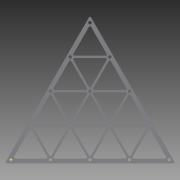
# Autodesk Inventor part: grid16-top
Saved by Autodesk Inventor 2013 (Build 170138000, 138)
## iProperties
Created: 2013-03-05
Part Number: grid16-top
Material: Generic
Document SubType Name: Modeling
Designer: Beth Scott
Density: 1 g/cm^3
Author: Beth Scott
Autodesk Inventor part; units mm, degrees
ref_plane "YZ Plane" through (0, 0, 0) normal (1, 0, 0) x (0, 1, 0)
ref_plane "XZ Plane" through (0, 0, 0) normal (0, 1, 0) x (-1, 0, 0)
ref_plane "XY Plane" through (0, 0, 0) normal (0, 0, 1) x (1, 0, 0)
sketch "Triangle 1mm" plane through (0, 0, 0) normal (0, 0, 1) x (1, 0, 0)
  line L0 (0, 0) -> (16.6665, 28.8672) construction
  line L1 (16.6665, 28.8672) -> (33.333, 0) construction
  line L2 (33.333, 0) -> (0, 0) construction
  line L3 (2.5981, 2.5) -> (15.8005, 25.3672)
  line L4 (17.5325, 25.3672) -> (30.7349, 2.5)
  line L5 (29.8689, 1) -> (3.4641, 1)
  arc A0 (17.5325, 25.3672) -> (15.8005, 25.3672) centre (16.6665, 24.8672) ccw
  arc A1 (29.8689, 1) -> (30.7349, 2.5) centre (29.8689, 2) ccw
  arc A2 (2.5981, 2.5) -> (3.4641, 1) centre (3.4641, 2) ccw
  line L6 (33.333, 0) -> (8.3332, 14.4336) construction
  line L7 (0, 0) -> (24.9997, 14.4336) construction
  line L8 (16.6665, 28.8672) -> (16.6665, 0) construction
  point P0 (16.9666, 9.7956)
  dimension "d14" = 33.333
  dimension "d17" = 1
  dimension "d18" = 1
  measures "d14" distance of L1.end L0.start
  measures "d17" radius of A2
  measures "d18" distance from line of L4 L7.end
sketch "Tri16 1mm" plane through (0, 0, 0) normal (0, 0, 1) x (1, 0, 0)
  line L0 (0, 0) -> (16.6665, 28.8672) construction
  line L1 (16.6665, 28.8672) -> (33.333, 0) construction
  line L2 (33.333, 0) -> (0, 0) construction
  line L3 (2.5981, 2.5) -> (15.8005, 25.3672)
  line L4 (17.5325, 25.3672) -> (30.7349, 2.5)
  line L5 (29.8689, 1) -> (3.4641, 1)
  arc A0 (17.5325, 25.3672) -> (15.8005, 25.3672) centre (16.6665, 24.8672) ccw
  arc A1 (29.8689, 1) -> (30.7349, 2.5) centre (29.8689, 2) ccw
  arc A2 (2.5981, 2.5) -> (3.4641, 1) centre (3.4641, 2) ccw
  line L6 (33.333, 0) -> (8.3333, 14.4336) construction
  line L7 (0, 0) -> (24.9998, 14.4336) construction
  line L8 (16.6665, 28.8672) -> (16.6665, 0) construction
  line L9 (33.333, 0) -> (49.9995, 28.8672) construction
  line L10 (49.9995, 28.8672) -> (66.666, 0) construction
  line L11 (66.666, 0) -> (33.333, 0) construction
  line L12 (35.9311, 2.5) -> (49.1335, 25.3672)
  line L13 (50.8655, 25.3672) -> (64.0679, 2.5)
  line L14 (63.2019, 1) -> (36.7971, 1)
  arc A3 (50.8655, 25.3672) -> (49.1335, 25.3672) centre (49.9995, 24.8672) ccw
  arc A4 (63.2019, 1) -> (64.0679, 2.5) centre (63.2019, 2) ccw
  arc A5 (35.9311, 2.5) -> (36.7971, 1) centre (36.7971, 2) ccw
  line L15 (66.666, 0) -> (41.6663, 14.4336) construction
  line L16 (33.333, 0) -> (58.3328, 14.4336) construction
  line L17 (49.9995, 28.8672) -> (49.9995, 0) construction
  line L18 (49.9995, 28.8672) -> (33.333, 0) construction
  line L19 (33.333, 0) -> (16.6665, 28.8672) construction
  line L20 (16.6665, 28.8672) -> (49.9995, 28.8672) construction
  line L21 (47.4014, 26.3672) -> (34.199, 3.5)
  line L22 (32.467, 3.5) -> (19.2646, 26.3672)
  line L23 (20.1306, 27.8672) -> (46.5354, 27.8672)
  arc A6 (32.467, 3.5) -> (34.199, 3.5) centre (33.333, 4) ccw
  arc A7 (20.1306, 27.8672) -> (19.2646, 26.3672) centre (20.1306, 26.8672) ccw
  arc A8 (47.4014, 26.3672) -> (46.5354, 27.8672) centre (46.5354, 26.8672) ccw
  line L24 (16.6665, 28.8672) -> (41.6663, 14.4336) construction
  line L25 (49.9995, 28.8672) -> (24.9998, 14.4336) construction
  line L26 (33.333, 0) -> (33.333, 28.8672) construction
  line L27 (83.3325, 28.8672) -> (66.666, 0) construction
  line L28 (66.666, 0) -> (49.9995, 28.8672) construction
  line L29 (49.9995, 28.8672) -> (83.3325, 28.8672) construction
  line L30 (80.7344, 26.3672) -> (67.532, 3.5)
  line L31 (65.8, 3.5) -> (52.5976, 26.3672)
  line L32 (53.4636, 27.8672) -> (79.8684, 27.8672)
  arc A9 (65.8, 3.5) -> (67.532, 3.5) centre (66.666, 4) ccw
  arc A10 (53.4636, 27.8672) -> (52.5976, 26.3672) centre (53.4636, 26.8672) ccw
  arc A11 (80.7344, 26.3672) -> (79.8684, 27.8672) centre (79.8684, 26.8672) ccw
  line L33 (49.9995, 28.8672) -> (74.9993, 14.4336) construction
  line L34 (83.3325, 28.8672) -> (58.3328, 14.4336) construction
  line L35 (66.666, 0) -> (66.666, 28.8672) construction
  line L36 (66.666, 0) -> (83.3325, 28.8672) construction
  line L37 (83.3325, 28.8672) -> (99.999, 0) construction
  line L38 (99.999, 0) -> (66.666, 0) construction
  line L39 (69.2641, 2.5) -> (82.4665, 25.3672)
  line L40 (84.1985, 25.3672) -> (97.4009, 2.5)
  line L41 (96.5349, 1) -> (70.1301, 1)
  arc A12 (84.1985, 25.3672) -> (82.4665, 25.3672) centre (83.3325, 24.8672) ccw
  arc A13 (96.5349, 1) -> (97.4009, 2.5) centre (96.5349, 2) ccw
  arc A14 (69.2641, 2.5) -> (70.1301, 1) centre (70.1301, 2) ccw
  line L42 (99.999, 0) -> (74.9993, 14.4336) construction
  line L43 (66.666, 0) -> (91.6658, 14.4336) construction
  line L44 (83.3325, 28.8672) -> (83.3325, 0) construction
  line L45 (99.999, 0) -> (116.6655, 28.8672) construction
  line L46 (116.6655, 28.8672) -> (133.332, 0) construction
  line L47 (133.332, 0) -> (99.999, 0) construction
  line L48 (102.5971, 2.5) -> (115.7995, 25.3672)
  line L49 (117.5315, 25.3672) -> (130.7339, 2.5)
  line L50 (129.8679, 1) -> (103.4631, 1)
  arc A15 (117.5315, 25.3672) -> (115.7995, 25.3672) centre (116.6655, 24.8672) ccw
  arc A16 (129.8679, 1) -> (130.7339, 2.5) centre (129.8679, 2) ccw
  arc A17 (102.5971, 2.5) -> (103.4631, 1) centre (103.4631, 2) ccw
  line L51 (133.332, 0) -> (108.3323, 14.4336) construction
  line L52 (99.999, 0) -> (124.9988, 14.4336) construction
  line L53 (116.6655, 28.8672) -> (116.6655, 0) construction
  line L54 (116.6655, 28.8672) -> (99.999, 0) construction
  line L55 (99.999, 0) -> (83.3325, 28.8672) construction
  line L56 (83.3325, 28.8672) -> (116.6655, 28.8672) construction
  line L57 (114.0674, 26.3672) -> (100.865, 3.5)
  line L58 (99.133, 3.5) -> (85.9306, 26.3672)
  line L59 (86.7966, 27.8672) -> (113.2014, 27.8672)
  arc A18 (99.133, 3.5) -> (100.865, 3.5) centre (99.999, 4) ccw
  arc A19 (86.7966, 27.8672) -> (85.9306, 26.3672) centre (86.7966, 26.8672) ccw
  arc A20 (114.0674, 26.3672) -> (113.2014, 27.8672) centre (113.2014, 26.8672) ccw
  line L60 (83.3325, 28.8672) -> (108.3323, 14.4336) construction
  line L61 (116.6655, 28.8672) -> (91.6658, 14.4336) construction
  line L62 (99.999, 0) -> (99.999, 28.8672) construction
  line L63 (16.6665, 28.8672) -> (33.333, 57.7344) construction
  line L64 (33.333, 57.7344) -> (49.9995, 28.8672) construction
  line L65 (49.9995, 28.8672) -> (16.6665, 28.8672) construction
  line L66 (19.2646, 31.3672) -> (32.467, 54.2344)
  line L67 (34.199, 54.2344) -> (47.4014, 31.3672)
  line L68 (46.5354, 29.8672) -> (20.1306, 29.8672)
  arc A21 (34.199, 54.2344) -> (32.467, 54.2344) centre (33.333, 53.7344) ccw
  arc A22 (46.5354, 29.8672) -> (47.4014, 31.3672) centre (46.5354, 30.8672) ccw
  arc A23 (19.2646, 31.3672) -> (20.1306, 29.8672) centre (20.1306, 30.8672) ccw
  line L69 (49.9995, 28.8672) -> (24.9998, 43.3008) construction
  line L70 (16.6665, 28.8672) -> (41.6663, 43.3008) construction
  line L71 (33.333, 57.7344) -> (33.333, 28.8672) construction
  line L72 (33.333, 57.7344) -> (49.9995, 86.6017) construction
  line L73 (49.9995, 86.6017) -> (66.666, 57.7344) construction
  line L74 (66.666, 57.7344) -> (33.333, 57.7344) construction
  line L75 (35.9311, 60.2344) -> (49.1335, 83.1017)
  line L76 (50.8655, 83.1017) -> (64.0679, 60.2344)
  line L77 (63.2019, 58.7344) -> (36.7971, 58.7344)
  arc A24 (50.8655, 83.1017) -> (49.1335, 83.1017) centre (49.9995, 82.6017) ccw
  arc A25 (63.2019, 58.7344) -> (64.0679, 60.2344) centre (63.2019, 59.7344) ccw
  arc A26 (35.9311, 60.2344) -> (36.7971, 58.7344) centre (36.7971, 59.7344) ccw
  line L78 (66.666, 57.7344) -> (41.6663, 72.1681) construction
  line L79 (33.333, 57.7344) -> (58.3328, 72.1681) construction
  line L80 (49.9995, 86.6017) -> (49.9995, 57.7344) construction
  line L81 (49.9995, 86.6017) -> (66.666, 115.4689) construction
  line L82 (66.666, 115.4689) -> (83.3325, 86.6017) construction
  line L83 (83.3325, 86.6017) -> (49.9995, 86.6017) construction
  line L84 (52.5976, 89.1017) -> (65.8, 111.9689)
  line L85 (67.532, 111.9689) -> (80.7344, 89.1017)
  line L86 (79.8684, 87.6017) -> (53.4636, 87.6017)
  arc A27 (67.532, 111.9689) -> (65.8, 111.9689) centre (66.666, 111.4689) ccw
  arc A28 (79.8684, 87.6017) -> (80.7344, 89.1017) centre (79.8684, 88.6017) ccw
  arc A29 (52.5976, 89.1017) -> (53.4636, 87.6017) centre (53.4636, 88.6017) ccw
  line L87 (83.3325, 86.6017) -> (58.3328, 101.0353) construction
  line L88 (49.9995, 86.6017) -> (74.9993, 101.0353) construction
  line L89 (66.666, 115.4689) -> (66.666, 86.6017) construction
  line L90 (66.666, 57.7344) -> (49.9995, 28.8672) construction
  line L91 (49.9995, 28.8672) -> (33.333, 57.7344) construction
  line L92 (33.333, 57.7344) -> (66.666, 57.7344) construction
  line L93 (64.0679, 55.2344) -> (50.8655, 32.3672)
  line L94 (49.1335, 32.3672) -> (35.9311, 55.2344)
  line L95 (36.7971, 56.7344) -> (63.2019, 56.7344)
  arc A30 (49.1335, 32.3672) -> (50.8655, 32.3672) centre (49.9995, 32.8672) ccw
  arc A31 (36.7971, 56.7344) -> (35.9311, 55.2344) centre (36.7971, 55.7344) ccw
  arc A32 (64.0679, 55.2344) -> (63.2019, 56.7344) centre (63.2019, 55.7344) ccw
  line L96 (33.333, 57.7344) -> (58.3328, 43.3008) construction
  line L97 (66.666, 57.7344) -> (41.6663, 43.3008) construction
  line L98 (49.9995, 28.8672) -> (49.9995, 57.7344) construction
  line L99 (83.3325, 86.6017) -> (66.666, 57.7344) construction
  line L100 (66.666, 57.7344) -> (49.9995, 86.6017) construction
  line L101 (49.9995, 86.6017) -> (83.3325, 86.6017) construction
  line L102 (80.7344, 84.1017) -> (67.532, 61.2344)
  line L103 (65.8, 61.2344) -> (52.5976, 84.1017)
  line L104 (53.4636, 85.6017) -> (79.8684, 85.6017)
  arc A33 (65.8, 61.2344) -> (67.532, 61.2344) centre (66.666, 61.7344) ccw
  arc A34 (53.4636, 85.6017) -> (52.5976, 84.1017) centre (53.4636, 84.6017) ccw
  arc A35 (80.7344, 84.1017) -> (79.8684, 85.6017) centre (79.8684, 84.6017) ccw
  line L105 (49.9995, 86.6017) -> (74.9993, 72.1681) construction
  line L106 (83.3325, 86.6017) -> (58.3328, 72.1681) construction
  line L107 (66.666, 57.7344) -> (66.666, 86.6017) construction
  line L108 (66.666, 57.7344) -> (83.3325, 86.6017) construction
  line L109 (83.3325, 86.6017) -> (99.999, 57.7344) construction
  line L110 (99.999, 57.7344) -> (66.666, 57.7344) construction
  line L111 (69.2641, 60.2344) -> (82.4665, 83.1017)
  line L112 (84.1985, 83.1017) -> (97.4009, 60.2344)
  line L113 (96.5349, 58.7344) -> (70.1301, 58.7344)
  arc A36 (84.1985, 83.1017) -> (82.4665, 83.1017) centre (83.3325, 82.6017) ccw
  arc A37 (96.5349, 58.7344) -> (97.4009, 60.2344) centre (96.5349, 59.7344) ccw
  arc A38 (69.2641, 60.2344) -> (70.1301, 58.7344) centre (70.1301, 59.7344) ccw
  line L114 (99.999, 57.7344) -> (74.9993, 72.1681) construction
  line L115 (66.666, 57.7344) -> (91.6658, 72.1681) construction
  line L116 (83.3325, 86.6017) -> (83.3325, 57.7344) construction
  line L117 (49.9995, 28.8672) -> (66.666, 57.7344) construction
  line L118 (66.666, 57.7344) -> (83.3325, 28.8672) construction
  line L119 (83.3325, 28.8672) -> (49.9995, 28.8672) construction
  line L120 (52.5976, 31.3672) -> (65.8, 54.2344)
  line L121 (67.532, 54.2344) -> (80.7344, 31.3672)
  line L122 (79.8684, 29.8672) -> (53.4636, 29.8672)
  arc A39 (67.532, 54.2344) -> (65.8, 54.2344) centre (66.666, 53.7344) ccw
  arc A40 (79.8684, 29.8672) -> (80.7344, 31.3672) centre (79.8684, 30.8672) ccw
  arc A41 (52.5976, 31.3672) -> (53.4636, 29.8672) centre (53.4636, 30.8672) ccw
  line L123 (83.3325, 28.8672) -> (58.3328, 43.3008) construction
  line L124 (49.9995, 28.8672) -> (74.9993, 43.3008) construction
  line L125 (66.666, 57.7344) -> (66.666, 28.8672) construction
  line L126 (83.3325, 28.8672) -> (99.999, 57.7344) construction
  line L127 (99.999, 57.7344) -> (116.6655, 28.8672) construction
  line L128 (116.6655, 28.8672) -> (83.3325, 28.8672) construction
  line L129 (85.9306, 31.3672) -> (99.133, 54.2344)
  line L130 (100.865, 54.2344) -> (114.0674, 31.3672)
  line L131 (113.2014, 29.8672) -> (86.7966, 29.8672)
  arc A42 (100.865, 54.2344) -> (99.133, 54.2344) centre (99.999, 53.7344) ccw
  arc A43 (113.2014, 29.8672) -> (114.0674, 31.3672) centre (113.2014, 30.8672) ccw
  arc A44 (85.9306, 31.3672) -> (86.7966, 29.8672) centre (86.7966, 30.8672) ccw
  line L132 (116.6655, 28.8672) -> (91.6658, 43.3008) construction
  line L133 (83.3325, 28.8672) -> (108.3323, 43.3008) construction
  line L134 (99.999, 57.7344) -> (99.999, 28.8672) construction
  line L135 (99.999, 57.7344) -> (83.3325, 28.8672) construction
  line L136 (83.3325, 28.8672) -> (66.666, 57.7344) construction
  line L137 (66.666, 57.7344) -> (99.999, 57.7344) construction
  line L138 (97.4009, 55.2344) -> (84.1985, 32.3672)
  line L139 (82.4665, 32.3672) -> (69.2641, 55.2344)
  line L140 (70.1301, 56.7344) -> (96.5349, 56.7344)
  arc A45 (82.4665, 32.3672) -> (84.1985, 32.3672) centre (83.3325, 32.8672) ccw
  arc A46 (70.1301, 56.7344) -> (69.2641, 55.2344) centre (70.1301, 55.7344) ccw
  arc A47 (97.4009, 55.2344) -> (96.5349, 56.7344) centre (96.5349, 55.7344) ccw
  line L141 (66.666, 57.7344) -> (91.6658, 43.3008) construction
  line L142 (99.999, 57.7344) -> (74.9993, 43.3008) construction
  line L143 (83.3325, 28.8672) -> (83.3325, 57.7344) construction
  point P0 (66.741, 38.5329)
sketch "Top Plate" plane through (0, 0, 0) normal (0, 1, 0) x (-1, 0, 0)
  line L0 (-4.3301, -1.5) -> (65.8, 119.9689)
  line L1 (67.532, 119.9689) -> (137.6621, -1.5)
  line L2 (-3.4641, -3) -> (136.7961, -3)
  circle A0 centre (33.333, 0) radius 1.5
  circle A1 centre (0, 0) radius 1.5
  circle A2 centre (16.6665, 28.8672) radius 1.5
  circle A3 centre (33.333, 57.7344) radius 1.5
  circle A4 centre (49.9995, 28.8672) radius 1.5
  circle A5 centre (66.666, 0) radius 1.5
  circle A6 centre (99.999, 0) radius 1.5
  circle A7 centre (133.332, 0) radius 1.5
  circle A8 centre (116.6655, 28.8672) radius 1.5
  circle A9 centre (99.999, 57.7344) radius 1.5
  circle A10 centre (83.3325, 28.8672) radius 1.5
  circle A11 centre (66.666, 57.7344) radius 1.5
  circle A12 centre (83.3325, 86.6017) radius 1.5
  circle A13 centre (49.9995, 86.6017) radius 1.5
  circle A14 centre (66.666, 115.4689) radius 1.5
  arc A15 (67.532, 119.9689) -> (65.8, 119.9689) centre (66.666, 119.4689) ccw
  arc A16 (136.7961, -3) -> (137.6621, -1.5) centre (136.7961, -2) ccw
  arc A17 (-4.3301, -1.5) -> (-3.4641, -3) centre (-3.4641, -2) ccw
  line L3 (0, 0) -> (-13.8976, -8.0238) construction
  line L4 (133.332, 0) -> (144.2364, -6.2956) construction
  line L5 (17.9655, 29.6172) -> (19.2646, 30.3672) construction
  line L6 (15.3675, 29.6172) -> (14.0684, 30.3672) construction
  line L7 (0, 0) -> (16.6665, 28.8672) construction
  line L8 (16.6665, 28.8672) -> (33.333, 0) construction
  line L9 (33.333, 0) -> (0, 0) construction
  line L10 (2.5981, 2.5) -> (15.8005, 25.3672)
  line L11 (17.5325, 25.3672) -> (30.7349, 2.5)
  line L12 (29.8689, 1) -> (3.4641, 1)
  arc A18 (17.5325, 25.3672) -> (15.8005, 25.3672) centre (16.6665, 24.8672) ccw
  arc A19 (29.8689, 1) -> (30.7349, 2.5) centre (29.8689, 2) ccw
  arc A20 (2.5981, 2.5) -> (3.4641, 1) centre (3.4641, 2) ccw
  line L13 (33.333, 0) -> (8.3333, 14.4336) construction
  line L14 (0, 0) -> (24.9998, 14.4336) construction
  line L15 (16.6665, 28.8672) -> (16.6665, 0) construction
  line L16 (33.333, 0) -> (49.9995, 28.8672) construction
  line L17 (49.9995, 28.8672) -> (66.666, 0) construction
  line L18 (66.666, 0) -> (33.333, 0) construction
  line L19 (35.9311, 2.5) -> (49.1335, 25.3672)
  line L20 (50.8655, 25.3672) -> (64.0679, 2.5)
  line L21 (63.2019, 1) -> (36.7971, 1)
  arc A21 (50.8655, 25.3672) -> (49.1335, 25.3672) centre (49.9995, 24.8672) ccw
  arc A22 (63.2019, 1) -> (64.0679, 2.5) centre (63.2019, 2) ccw
  arc A23 (35.9311, 2.5) -> (36.7971, 1) centre (36.7971, 2) ccw
  line L22 (66.666, 0) -> (41.6663, 14.4336) construction
  line L23 (33.333, 0) -> (58.3328, 14.4336) construction
  line L24 (49.9995, 28.8672) -> (49.9995, 0) construction
  line L25 (49.9995, 28.8672) -> (33.333, 0) construction
  line L26 (33.333, 0) -> (16.6665, 28.8672) construction
  line L27 (16.6665, 28.8672) -> (49.9995, 28.8672) construction
  line L28 (47.4014, 26.3672) -> (34.199, 3.5)
  line L29 (32.467, 3.5) -> (19.2646, 26.3672)
  line L30 (20.1306, 27.8672) -> (46.5354, 27.8672)
  arc A24 (32.467, 3.5) -> (34.199, 3.5) centre (33.333, 4) ccw
  arc A25 (20.1306, 27.8672) -> (19.2646, 26.3672) centre (20.1306, 26.8672) ccw
  arc A26 (47.4014, 26.3672) -> (46.5354, 27.8672) centre (46.5354, 26.8672) ccw
  line L31 (16.6665, 28.8672) -> (41.6663, 14.4336) construction
  line L32 (49.9995, 28.8672) -> (24.9998, 14.4336) construction
  line L33 (33.333, 0) -> (33.333, 28.8672) construction
  line L34 (83.3325, 28.8672) -> (66.666, 0) construction
  line L35 (66.666, 0) -> (49.9995, 28.8672) construction
  line L36 (49.9995, 28.8672) -> (83.3325, 28.8672) construction
  line L37 (80.7344, 26.3672) -> (67.532, 3.5)
  line L38 (65.8, 3.5) -> (52.5976, 26.3672)
  line L39 (53.4636, 27.8672) -> (79.8684, 27.8672)
  arc A27 (65.8, 3.5) -> (67.532, 3.5) centre (66.666, 4) ccw
  arc A28 (53.4636, 27.8672) -> (52.5976, 26.3672) centre (53.4636, 26.8672) ccw
  arc A29 (80.7344, 26.3672) -> (79.8684, 27.8672) centre (79.8684, 26.8672) ccw
  line L40 (49.9995, 28.8672) -> (74.9993, 14.4336) construction
  line L41 (83.3325, 28.8672) -> (58.3328, 14.4336) construction
  line L42 (66.666, 0) -> (66.666, 28.8672) construction
  line L43 (66.666, 0) -> (83.3325, 28.8672) construction
  line L44 (83.3325, 28.8672) -> (99.999, 0) construction
  line L45 (99.999, 0) -> (66.666, 0) construction
  line L46 (69.2641, 2.5) -> (82.4665, 25.3672)
  line L47 (84.1985, 25.3672) -> (97.4009, 2.5)
  line L48 (96.5349, 1) -> (70.1301, 1)
  arc A30 (84.1985, 25.3672) -> (82.4665, 25.3672) centre (83.3325, 24.8672) ccw
  arc A31 (96.5349, 1) -> (97.4009, 2.5) centre (96.5349, 2) ccw
  arc A32 (69.2641, 2.5) -> (70.1301, 1) centre (70.1301, 2) ccw
  line L49 (99.999, 0) -> (74.9993, 14.4336) construction
  line L50 (66.666, 0) -> (91.6658, 14.4336) construction
  line L51 (83.3325, 28.8672) -> (83.3325, 0) construction
  line L52 (99.999, 0) -> (116.6655, 28.8672) construction
  line L53 (116.6655, 28.8672) -> (133.332, 0) construction
  line L54 (133.332, 0) -> (99.999, 0) construction
  line L55 (102.5971, 2.5) -> (115.7995, 25.3672)
  line L56 (117.5315, 25.3672) -> (130.7339, 2.5)
  line L57 (129.8679, 1) -> (103.4631, 1)
  arc A33 (117.5315, 25.3672) -> (115.7995, 25.3672) centre (116.6655, 24.8672) ccw
  arc A34 (129.8679, 1) -> (130.7339, 2.5) centre (129.8679, 2) ccw
  arc A35 (102.5971, 2.5) -> (103.4631, 1) centre (103.4631, 2) ccw
  line L58 (133.332, 0) -> (108.3323, 14.4336) construction
  line L59 (99.999, 0) -> (124.9988, 14.4336) construction
  line L60 (116.6655, 28.8672) -> (116.6655, 0) construction
  line L61 (116.6655, 28.8672) -> (99.999, 0) construction
  line L62 (99.999, 0) -> (83.3325, 28.8672) construction
  line L63 (83.3325, 28.8672) -> (116.6655, 28.8672) construction
  line L64 (114.0674, 26.3672) -> (100.865, 3.5)
  line L65 (99.133, 3.5) -> (85.9306, 26.3672)
  line L66 (86.7966, 27.8672) -> (113.2014, 27.8672)
  arc A36 (99.133, 3.5) -> (100.865, 3.5) centre (99.999, 4) ccw
  arc A37 (86.7966, 27.8672) -> (85.9306, 26.3672) centre (86.7966, 26.8672) ccw
  arc A38 (114.0674, 26.3672) -> (113.2014, 27.8672) centre (113.2014, 26.8672) ccw
  line L67 (83.3325, 28.8672) -> (108.3323, 14.4336) construction
  line L68 (116.6655, 28.8672) -> (91.6658, 14.4336) construction
  line L69 (99.999, 0) -> (99.999, 28.8672) construction
  line L70 (16.6665, 28.8672) -> (33.333, 57.7344) construction
  line L71 (33.333, 57.7344) -> (49.9995, 28.8672) construction
  line L72 (49.9995, 28.8672) -> (16.6665, 28.8672) construction
  line L73 (19.2646, 31.3672) -> (32.467, 54.2344)
  line L74 (34.199, 54.2344) -> (47.4014, 31.3672)
  line L75 (46.5354, 29.8672) -> (20.1306, 29.8672)
  arc A39 (34.199, 54.2344) -> (32.467, 54.2344) centre (33.333, 53.7344) ccw
  arc A40 (46.5354, 29.8672) -> (47.4014, 31.3672) centre (46.5354, 30.8672) ccw
  arc A41 (19.2646, 31.3672) -> (20.1306, 29.8672) centre (20.1306, 30.8672) ccw
  line L76 (49.9995, 28.8672) -> (24.9998, 43.3008) construction
  line L77 (16.6665, 28.8672) -> (41.6663, 43.3008) construction
  line L78 (33.333, 57.7344) -> (33.333, 28.8672) construction
  line L79 (33.333, 57.7344) -> (49.9995, 86.6017) construction
  line L80 (49.9995, 86.6017) -> (66.666, 57.7344) construction
  line L81 (66.666, 57.7344) -> (33.333, 57.7344) construction
  line L82 (35.9311, 60.2344) -> (49.1335, 83.1017)
  line L83 (50.8655, 83.1017) -> (64.0679, 60.2344)
  line L84 (63.2019, 58.7344) -> (36.7971, 58.7344)
  arc A42 (50.8655, 83.1017) -> (49.1335, 83.1017) centre (49.9995, 82.6017) ccw
  arc A43 (63.2019, 58.7344) -> (64.0679, 60.2344) centre (63.2019, 59.7344) ccw
  arc A44 (35.9311, 60.2344) -> (36.7971, 58.7344) centre (36.7971, 59.7344) ccw
  line L85 (66.666, 57.7344) -> (41.6663, 72.1681) construction
  line L86 (33.333, 57.7344) -> (58.3328, 72.1681) construction
  line L87 (49.9995, 86.6017) -> (49.9995, 57.7344) construction
  line L88 (49.9995, 86.6017) -> (66.666, 115.4689) construction
  line L89 (66.666, 115.4689) -> (83.3325, 86.6017) construction
  line L90 (83.3325, 86.6017) -> (49.9995, 86.6017) construction
  line L91 (52.5976, 89.1017) -> (65.8, 111.9689)
  line L92 (67.532, 111.9689) -> (80.7344, 89.1017)
  line L93 (79.8684, 87.6017) -> (53.4636, 87.6017)
  arc A45 (67.532, 111.9689) -> (65.8, 111.9689) centre (66.666, 111.4689) ccw
  arc A46 (79.8684, 87.6017) -> (80.7344, 89.1017) centre (79.8684, 88.6017) ccw
  arc A47 (52.5976, 89.1017) -> (53.4636, 87.6017) centre (53.4636, 88.6017) ccw
  line L94 (83.3325, 86.6017) -> (58.3328, 101.0353) construction
  line L95 (49.9995, 86.6017) -> (74.9993, 101.0353) construction
  line L96 (66.666, 115.4689) -> (66.666, 86.6017) construction
  line L97 (66.666, 57.7344) -> (49.9995, 28.8672) construction
  line L98 (49.9995, 28.8672) -> (33.333, 57.7344) construction
  line L99 (33.333, 57.7344) -> (66.666, 57.7344) construction
  line L100 (64.0679, 55.2344) -> (50.8655, 32.3672)
  line L101 (49.1335, 32.3672) -> (35.9311, 55.2344)
  line L102 (36.7971, 56.7344) -> (63.2019, 56.7344)
  arc A48 (49.1335, 32.3672) -> (50.8655, 32.3672) centre (49.9995, 32.8672) ccw
  arc A49 (36.7971, 56.7344) -> (35.9311, 55.2344) centre (36.7971, 55.7344) ccw
  arc A50 (64.0679, 55.2344) -> (63.2019, 56.7344) centre (63.2019, 55.7344) ccw
  line L103 (33.333, 57.7344) -> (58.3328, 43.3008) construction
  line L104 (66.666, 57.7344) -> (41.6663, 43.3008) construction
  line L105 (49.9995, 28.8672) -> (49.9995, 57.7344) construction
  line L106 (83.3325, 86.6017) -> (66.666, 57.7344) construction
  line L107 (66.666, 57.7344) -> (49.9995, 86.6017) construction
  line L108 (49.9995, 86.6017) -> (83.3325, 86.6017) construction
  line L109 (80.7344, 84.1017) -> (67.532, 61.2344)
  line L110 (65.8, 61.2344) -> (52.5976, 84.1017)
  line L111 (53.4636, 85.6017) -> (79.8684, 85.6017)
  arc A51 (65.8, 61.2344) -> (67.532, 61.2344) centre (66.666, 61.7344) ccw
  arc A52 (53.4636, 85.6017) -> (52.5976, 84.1017) centre (53.4636, 84.6017) ccw
  arc A53 (80.7344, 84.1017) -> (79.8684, 85.6017) centre (79.8684, 84.6017) ccw
  line L112 (49.9995, 86.6017) -> (74.9993, 72.1681) construction
  line L113 (83.3325, 86.6017) -> (58.3328, 72.1681) construction
  line L114 (66.666, 57.7344) -> (66.666, 86.6017) construction
  line L115 (66.666, 57.7344) -> (83.3325, 86.6017) construction
  line L116 (83.3325, 86.6017) -> (99.999, 57.7344) construction
  line L117 (99.999, 57.7344) -> (66.666, 57.7344) construction
  line L118 (69.2641, 60.2344) -> (82.4665, 83.1017)
  line L119 (84.1985, 83.1017) -> (97.4009, 60.2344)
  line L120 (96.5349, 58.7344) -> (70.1301, 58.7344)
  arc A54 (84.1985, 83.1017) -> (82.4665, 83.1017) centre (83.3325, 82.6017) ccw
  arc A55 (96.5349, 58.7344) -> (97.4009, 60.2344) centre (96.5349, 59.7344) ccw
  arc A56 (69.2641, 60.2344) -> (70.1301, 58.7344) centre (70.1301, 59.7344) ccw
  line L121 (99.999, 57.7344) -> (74.9993, 72.1681) construction
  line L122 (66.666, 57.7344) -> (91.6658, 72.1681) construction
  line L123 (83.3325, 86.6017) -> (83.3325, 57.7344) construction
  line L124 (49.9995, 28.8672) -> (66.666, 57.7344) construction
  line L125 (66.666, 57.7344) -> (83.3325, 28.8672) construction
  line L126 (83.3325, 28.8672) -> (49.9995, 28.8672) construction
  line L127 (52.5976, 31.3672) -> (65.8, 54.2344)
  line L128 (67.532, 54.2344) -> (80.7344, 31.3672)
  line L129 (79.8684, 29.8672) -> (53.4636, 29.8672)
  arc A57 (67.532, 54.2344) -> (65.8, 54.2344) centre (66.666, 53.7344) ccw
  arc A58 (79.8684, 29.8672) -> (80.7344, 31.3672) centre (79.8684, 30.8672) ccw
  arc A59 (52.5976, 31.3672) -> (53.4636, 29.8672) centre (53.4636, 30.8672) ccw
  line L130 (83.3325, 28.8672) -> (58.3328, 43.3008) construction
  line L131 (49.9995, 28.8672) -> (74.9993, 43.3008) construction
  line L132 (66.666, 57.7344) -> (66.666, 28.8672) construction
  line L133 (83.3325, 28.8672) -> (99.999, 57.7344) construction
  line L134 (99.999, 57.7344) -> (116.6655, 28.8672) construction
  line L135 (116.6655, 28.8672) -> (83.3325, 28.8672) construction
  line L136 (85.9306, 31.3672) -> (99.133, 54.2344)
  line L137 (100.865, 54.2344) -> (114.0674, 31.3672)
  line L138 (113.2014, 29.8672) -> (86.7966, 29.8672)
  arc A60 (100.865, 54.2344) -> (99.133, 54.2344) centre (99.999, 53.7344) ccw
  arc A61 (113.2014, 29.8672) -> (114.0674, 31.3672) centre (113.2014, 30.8672) ccw
  arc A62 (85.9306, 31.3672) -> (86.7966, 29.8672) centre (86.7966, 30.8672) ccw
  line L139 (116.6655, 28.8672) -> (91.6658, 43.3008) construction
  line L140 (83.3325, 28.8672) -> (108.3323, 43.3008) construction
  line L141 (99.999, 57.7344) -> (99.999, 28.8672) construction
  line L142 (99.999, 57.7344) -> (83.3325, 28.8672) construction
  line L143 (83.3325, 28.8672) -> (66.666, 57.7344) construction
  line L144 (66.666, 57.7344) -> (99.999, 57.7344) construction
  line L145 (97.4009, 55.2344) -> (84.1985, 32.3672)
  line L146 (82.4665, 32.3672) -> (69.2641, 55.2344)
  line L147 (70.1301, 56.7344) -> (96.5349, 56.7344)
  arc A63 (82.4665, 32.3672) -> (84.1985, 32.3672) centre (83.3325, 32.8672) ccw
  arc A64 (70.1301, 56.7344) -> (69.2641, 55.2344) centre (70.1301, 55.7344) ccw
  arc A65 (97.4009, 55.2344) -> (96.5349, 56.7344) centre (96.5349, 55.7344) ccw
  line L148 (66.666, 57.7344) -> (91.6658, 43.3008) construction
  line L149 (99.999, 57.7344) -> (74.9993, 43.3008) construction
  line L150 (83.3325, 28.8672) -> (83.3325, 57.7344) construction
  dimension "d25" = 3
  constraints: 18 centre point, 14 end point, 14 equal radius, 8 point on circle, 6 tangent, 3 point on line, 1 equal length, 1 horizontal, 1 perpendicular, 26 other
  measures "d25" diameter of A0
extrude "Top Plate extrusion" add sketch "Top Plate" along normal blind 1.5875
sketch "LED Strip" plane through (0, 0, 0) normal (0, 1, 0) x (-1, 0, 0)
  point P0 (0, 0)
body "Solid2"
